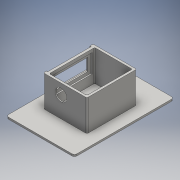
# Autodesk Inventor part: sampleChamberExt
Saved by Autodesk Inventor 2016 (Build 200138000, 138)
## iProperties
Created: 2016-11-02
Part Number: sampleChamberExt
Material: Generic
Document SubType Name: Modeling
Designer: sims01
Density: 1 g/cm^3
Appearance: Default
Author: sims01
Autodesk Inventor part; units mm, degrees
ref_plane "YZ Plane" through (0, 0, 0) normal (1, 0, 0) x (0, 1, 0)
ref_plane "XZ Plane" through (0, 0, 0) normal (0, 1, 0) x (-1, 0, 0)
ref_plane "XY Plane" through (0, 0, 0) normal (0, 0, 1) x (1, 0, 0)
sketch "Sketch1" plane through (0, 0, 0) normal (0, 0, 1) x (1, 0, 0)
  line L0 (-50.875, 79.875) -> (50.875, 79.875)
  line L1 (54.875, 75.875) -> (54.875, -75.875)
  line L2 (50.875, -79.875) -> (-50.875, -79.875)
  line L3 (-54.875, -75.875) -> (-54.875, 75.875)
  arc A0 (-50.875, 79.875) -> (-54.875, 75.875) centre (-50.875, 75.875) ccw
  arc A1 (54.875, 75.875) -> (50.875, 79.875) centre (50.875, 75.875) ccw
  arc A2 (-54.875, -75.875) -> (-50.875, -79.875) centre (-50.875, -75.875) ccw
  arc A3 (50.875, -79.875) -> (54.875, -75.875) centre (50.875, -75.875) ccw
  point P0 (0, 0)
  point P1 (-54.875, 79.875)
  point P2 (-54.875, -79.875)
  dimension "d0" = 159.75
  dimension "d1" = 79.875
  dimension "d2" = 109.75
  dimension "d3" = 4
  dimension "d6" = 54.875
  constraints: 8 end point, 8 point on circle, 8 tangent, 4 centre point, 4 point on line, 3 equal radius, 2 parallel, 1 horizontal, 1 perpendicular
  measures "d0" distance of point (-54.875, -79.875) point (-54.875, 79.875)
  measures "d1" distance from line of point (0, 0) L0
  measures "d2" distance between parallel lines of L1 L3
  measures "d3" radius of A0
  measures "d6" distance from line of point (0, 0) L1
extrude "xyAttach" add sketch "Sketch1" along normal blind 3
sketch "Sketch2" plane through (0, 0, 3) normal (0, 0, 1) x (1, 0, 0)
  line L0 (-33, 40) -> (33, 40)
  line L1 (35, 38) -> (35, -38)
  line L2 (33, -40) -> (-33, -40)
  line L3 (-35, -38) -> (-35, 38)
  line L4 (-27, 36.5) -> (29.5, 36.5)
  line L5 (31.5, 34.5) -> (31.5, -34.5)
  line L6 (29.5, -36.5) -> (-27, -36.5)
  line L7 (-29, -34.5) -> (-29, 34.5)
  arc A0 (-33, 40) -> (-35, 38) centre (-33, 38) ccw
  arc A1 (-35, -38) -> (-33, -40) centre (-33, -38) ccw
  arc A2 (33, -40) -> (35, -38) centre (33, -38) ccw
  arc A3 (35, 38) -> (33, 40) centre (33, 38) ccw
  arc A4 (31.5, 34.5) -> (29.5, 36.5) centre (29.5, 34.5) ccw
  arc A5 (29.5, -36.5) -> (31.5, -34.5) centre (29.5, -34.5) ccw
  arc A6 (-29, -34.5) -> (-27, -36.5) centre (-27, -34.5) ccw
  arc A7 (-27, 36.5) -> (-29, 34.5) centre (-27, 34.5) ccw
  point P0 (0, 0)
  point P1 (35, -40)
  point P2 (35, 40)
  point P3 (-35, -40)
  dimension "d7" = 70
  dimension "d8" = 80
  dimension "d9" = 40
  dimension "d10" = 35
  dimension "d11" = 3.5
  dimension "d12" = 3.5
  dimension "d13" = 3.5
  dimension "d14" = 6
  dimension "d15" = 2
  constraints: 16 end point, 16 point on circle, 16 tangent, 8 centre point, 7 equal radius, 6 point on line, 4 parallel, 2 horizontal, 2 perpendicular
  measures "d7" distance of point (35, -40) point (-35, -40)
  measures "d8" distance of point (35, 40) point (35, -40)
  measures "d9" distance from line of point (0, 0) L0
  measures "d10" distance from line of point (0, 0) L1
  measures "d11" distance between parallel lines of L4 L0
  measures "d12" distance between parallel lines of L1 L5
  measures "d13" distance between parallel lines of L2 L6
  measures "d14" distance between parallel lines of L3 L7
  measures "d15" radius of A0
extrude "chamberExtrusion" add sketch "Sketch2" along normal blind 50
sketch "Sketch3" plane through (0, 0, 3) normal (0, 0, 1) x (1, 0, 0)
  circle A0 centre (15, 0) radius 2.825
  circle A1 centre (0, 15) radius 2.825
  circle A2 centre (0, 0) radius 2.825
  circle A3 centre (-15, 0) radius 2.825
  circle A4 centre (0, -15) radius 2.825
  dimension "d18" = 5.65
  dimension "d19" = 5.65
  dimension "d20" = 5.65
  dimension "d21" = 5.65
  dimension "d22" = 5.65
  dimension "d23" = 15
  dimension "d24" = 15
  dimension "d25" = 15
  dimension "d26" = 15
  constraints: 5 centre point, 2 coincident, 2 horizontal alignment, 2 vertical alignment
  measures "d18" diameter of A1
  measures "d19" diameter of A0
  measures "d20" diameter of A2
  measures "d21" diameter of A3
  measures "d22" diameter of A4
  measures "d23" distance of point (0, 0) A1.centre
  measures "d24" distance of A0.centre point (0, 0)
  measures "d25" distance of A4.centre point (0, 0)
  measures "d26" distance of A3.centre point (0, 0)
extrude "magnetsExtrusion" cut sketch "Sketch3" against normal blind 2.75
sketch "Sketch5" plane through (-29, -34.5, 3) normal (1, 0, 0) x (0, 0, -1)
  line L0 (-45, 2) -> (-15, 2)
  line L1 (-15, 2) -> (-15, 67)
  line L2 (-15, 67) -> (-45, 67)
  line L3 (-45, 67) -> (-45, 2)
  line L4 (0, 69) -> (0, 0) projected
  point P0 (3, 34.5)
  dimension "d29" = 65
  dimension "d30" = 30
  dimension "d31" = 32.5
  dimension "d32" = 45
  constraints: 8 end point, 2 parallel, 1 horizontal, 1 perpendicular
  measures "d29" distance of L2.end L0.start
  measures "d30" distance of L1.end L2.end
  measures "d31" distance from line of point (3, 34.5) L0
  measures "d32" distance between parallel lines of L4 L3
extrude "coverSlipMountExt" cut sketch "Sketch5" against normal blind 2
sketch "Sketch6" plane through (-31, -34.5, 3) normal (1, 0, 0) x (0, 0, -1)
  line L0 (-40, 7) -> (-20, 7)
  line L1 (-20, 7) -> (-20, 62)
  line L2 (-20, 62) -> (-40, 62)
  line L3 (-40, 62) -> (-40, 7)
  line L4 (0, 69) -> (0, 0) projected
  point P0 (3, 34.5)
  dimension "d35" = 55
  dimension "d36" = 20
  dimension "d37" = 27.5
  dimension "d38" = 40
  constraints: 8 end point, 2 parallel, 1 horizontal, 1 perpendicular
  measures "d35" distance of L2.end L0.start
  measures "d36" distance of L1.end L2.end
  measures "d37" distance from line of point (3, 34.5) L2
  measures "d38" distance between parallel lines of L4 L3
extrude "coverSlipWindowExt" cut sketch "Sketch6" against normal up to surface (4 mm away)
sketch "Sketch7" plane through (-35, -38, 3) normal (-1, 0, 0) x (0, 0, 1)
  line L0 (50, 73) -> (0, 73)
  line L1 (0, 73) -> (0, 3)
  line L2 (0, 3) -> (50, 3)
  line L3 (50, 3) -> (50, 73)
  line L4 (50, 76) -> (50, 0) projected
  line L5 (0, 0) -> (0, 76) projected
  point P0 (-3, 38)
  dimension "d41" = 70
  dimension "d42" = 35
  constraints: 8 end point, 2 collinear, 2 parallel, 1 horizontal, 1 perpendicular
  measures "d41" distance of L2.end L0.start
  measures "d42" distance from line of L2 point (-3, 38)
extrude "illObjExt" cut sketch "Sketch7" against normal blind 2
sketch "Sketch8" plane through (-27, -36.5, 3) normal (0, 1, 0) x (1, 0, 0)
  circle A0 centre (20.5, -33.5) radius 12.5
  point P0 (27, 3)
  point P1 (-2, -50)
  point P2 (-8, -50)
  point P3 (-6, -50)
  dimension "d45" = 25
  dimension "d53" = 26.5
  constraints: 1 centre point
  measures "d45" diameter of A0
  measures "d53" horizontal distance of point (-6, -50) A0.centre
extrude "circCovSlipMount" cut sketch "Sketch8" against normal blind 2
sketch "Sketch9" plane through (-6.5, -38.5, 36.5) normal (0, 1, 0) x (1, 0, 0)
  circle A0 centre (0, 0) radius 9.5
  circle A1 centre (0, 0) radius 12.5 projected
  point P0 (6.5, 36.5)
  dimension "d50" = 19
  constraints: 1 centre point, 1 concentric
  measures "d50" diameter of A0
extrude "circCovSlipWindowExt" cut sketch "Sketch9" against normal up to surface (1.5 mm away) contours A0
equation "\"d1\" = 0.5 * d0"
equation "\"d6\" = 0.5 * d2"
equation "\"d9\" = 0.5 * d8"
equation "\"d10\" = 0.5 * d7"
equation "\"d12\" = d11"
equation "\"d13\" = d11"
equation "\"d19\" = d18"
equation "\"d20\" = d19"
equation "\"d21\" = d20"
equation "\"d22\" = d21"
equation "\"d24\" = d23"
equation "\"d25\" = d23"
equation "\"d26\" = d23"
equation "\"d31\" = 0.5 * d29"
equation "\"d37\" = 0.5 * d35"
equation "\"d42\" = 0.5 * d41"
body "Solid1"
